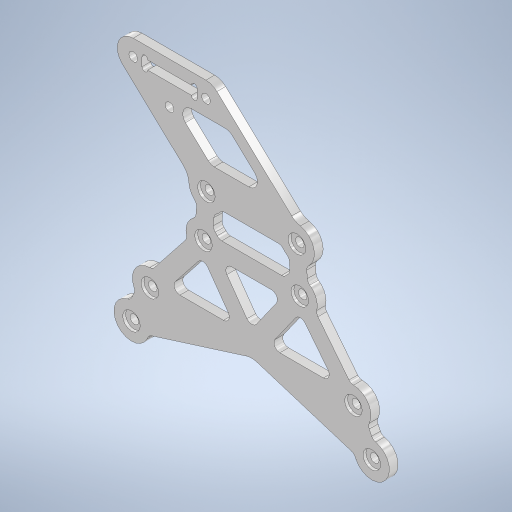
# Autodesk Inventor part: 中間ユニット外(shin)
Saved by Autodesk Inventor 2023 (Build 270158030, 158C)
## iProperties
Created: 2022-05-12
Part Number: 中間ユニット外(shin)
Material: アルミニウム 2014-T6
Document SubType Name: Modeling
Designer: muzho
Density: 2.78927 g/cm^3
Appearance: サテン
Author: muzho
Autodesk Inventor part; units mm, degrees
ref_plane "YZ Plane" through (0, 0, 0) normal (1, 0, 0) x (0, 1, 0)
ref_plane "XZ Plane" through (0, 0, 0) normal (0, 1, 0) x (-1, 0, 0)
ref_plane "XY Plane" through (0, 0, 0) normal (0, 0, 1) x (1, 0, 0)
sketch "スケッチ1" plane through (0, 0, 0) normal (0, 0, 1) x (1, 0, 0)
  circle A0 centre (-15.5646, 38.363) radius 1.5
  circle A1 centre (-15.5646, 38.363) radius 3.025
  circle A2 centre (-16.5506, 23.3453) radius 1.5
  circle A3 centre (-16.5506, 23.3453) radius 3.025
  circle A4 centre (-35, 0) radius 1.5
  circle A5 centre (-35, 0) radius 3.025
  circle A6 centre (-41.3199, -13) radius 1.5
  circle A7 centre (-41.3199, -13) radius 3.025
  circle A8 centre (41.3199, -13) radius 1.5
  circle A9 centre (41.3199, -13) radius 3.025
  circle A10 centre (35, 0) radius 3.025
  circle A11 centre (35, 0) radius 1.5
  circle A12 centre (16.5506, 23.3453) radius 3.025
  circle A13 centre (16.5506, 23.3453) radius 1.5
  circle A14 centre (15.5646, 38.363) radius 3.025
  circle A15 centre (15.5646, 38.363) radius 1.5
  circle A16 centre (-15.5646, 38.363) radius 6.025
  circle A17 centre (-16.5506, 23.3453) radius 6.025
  circle A18 centre (-35, 0) radius 6.025
  circle A19 centre (-41.3199, -13) radius 6.025
  circle A20 centre (15.5646, 38.363) radius 6.025
  circle A21 centre (16.5506, 23.3453) radius 6.025
  circle A22 centre (35, 0) radius 6.025
  circle A23 centre (41.3199, -13) radius 6.025
  line L0 (15.5646, 38.363) -> (16.5506, 23.3453) construction
  line L1 (16.5506, 23.3453) -> (35, 0) construction
  line L2 (35, 0) -> (41.3199, -13) construction
  line L3 (12.9134, 32.9527) -> (13.2147, 28.3626)
  line L4 (18.9005, 33.3458) -> (19.2019, 28.7557)
  line L5 (17.4366, 17.3858) -> (28.8054, 3)
  line L6 (22.144, 21.106) -> (34.114, 5.9595)
  line L7 (39.9825, -3.3875) -> (41.7335, -6.9892)
  line L8 (15.5646, 38.363) -> (0, 38.363) construction
  line L9 (16.5506, 23.3453) -> (0, 23.3453) construction
  line L10 (16.5506, 23.3453) -> (0, 0) construction
  line L11 (0, 0) -> (35, 0) construction
  line L12 (41.3199, -13) -> (0, 0) construction
  line L13 (10.3396, 41.363) -> (0, 41.363)
  line L14 (10.3396, 35.363) -> (0, 35.363)
  line L15 (11.3256, 26.3453) -> (0, 26.3453)
  line L16 (10.7463, 20.3453) -> (0, 20.3453)
  line L17 (10.7463, 20.3453) -> (-0.0011, 5.1857)
  line L18 (15.9761, 17.3478) -> (5.8043, 3)
  line L19 (5.8043, 3) -> (28.8054, 3)
  line L20 (28.8054, 3) -> (29.4066, 2.2393) construction
  line L21 (28.8054, 3) -> (29.775, 3) construction
  line L22 (29.5814, -2.6342) -> (35.9013, -15.6342)
  line L23 (29.7592, -3) -> (19.5315, -3)
  line L24 (19.5315, -3) -> (31.606, -6.7989)
  line L25 (1.8007, -3.7115) -> (35.216, -14.2246)
  line L26 (0, 0) -> (0, 9.2146) construction
  line L27 (-10.3396, 41.363) -> (0, 41.363)
  line L28 (-10.3396, 35.363) -> (0, 35.363)
  line L29 (-11.3256, 26.3453) -> (0, 26.3453)
  line L30 (-10.7463, 20.3453) -> (0, 20.3453)
  line L31 (-12.9134, 32.9527) -> (-13.2147, 28.3626)
  line L32 (-18.9005, 33.3458) -> (-19.2019, 28.7557)
  line L33 (-10.7463, 20.3453) -> (0.0011, 5.1857)
  line L34 (-15.9761, 17.3478) -> (-5.8043, 3)
  line L35 (-17.4366, 17.3858) -> (-28.8054, 3)
  line L36 (-22.144, 21.106) -> (-34.114, 5.9595)
  line L37 (-5.8043, 3) -> (-28.8054, 3)
  line L38 (-29.7592, -3) -> (-19.5315, -3)
  line L39 (-19.5315, -3) -> (-31.606, -6.7989)
  line L40 (-29.5814, -2.6342) -> (-35.9013, -15.6342)
  line L41 (-39.9825, -3.3875) -> (-41.7335, -6.9892)
  line L42 (-1.8007, -3.7115) -> (-35.216, -14.2246)
  arc A24 (1.8007, -3.7115) -> (-1.8007, -3.7115) centre (0, -9.4349) ccw
  point P0 (0, 5.1872)
  point P1 (-35.9013, -15.6342)
  point P2 (0, -3.145)
  dimension "d0" = 3
  dimension "d1" = 3
  dimension "d2" = 3
  dimension "d3" = 3
  dimension "d4" = 3
  dimension "d5" = 3
  dimension "d6" = 3
  dimension "d7" = 3
  dimension "d8" = 6
  dimension "d9" = 3
  dimension "d10" = 6
  dimension "d11" = 3
  dimension "d12" = 6
  dimension "d13" = 3
  dimension "d14" = 6
  dimension "d15" = 3
  dimension "d16" = 6
  dimension "d17" = 3
  dimension "d18" = 3
  dimension "d19" = 3
  dimension "d20" = 6
  dimension "d21" = 3
  dimension "d22" = 3
  dimension "d57" = 6
  constraints: 88 end point, 25 centre point, 24 symmetric about line, 19 point on circle, 10 horizontal, 10 parallel, 6 point on line, 3 tangent, 1 vertical, 25 other
  measures "d0" radial gap between concentric circles of A1 A16
  measures "d1" radial gap between concentric circles of A3 A17
  measures "d2" radial gap between concentric circles of A5 A18
  measures "d3" radial gap between concentric circles of A7 A19
  measures "d4" radial gap between concentric circles of A14 A20
  measures "d5" radial gap between concentric circles of A12 A21
  measures "d6" radial gap between concentric circles of A10 A22
  measures "d7" radial gap between concentric circles of A9 A23
  measures "d8" distance between parallel lines of L3 L4
  measures "d9" distance between parallel lines of L3 L0
  measures "d10" distance between parallel lines of L5 L6
  measures "d11" distance between parallel lines of L5 L1
  measures "d12" distance between parallel lines of L14 L13
  measures "d13" distance between parallel lines of L14 L8
  measures "d14" distance between parallel lines of L16 L15
  measures "d15" distance between parallel lines of L16 L9
  measures "d16" distance between parallel lines of L18 L17
  measures "d17" distance between parallel lines of L17 L10
  measures "d18" distance between parallel lines of L11 L19
  measures "d19" distance between parallel lines of L2 L7
  measures "d20" distance between parallel lines of L19 L23
  measures "d21" distance between parallel lines of L12 L24
  measures "d22" distance between parallel lines of L25 L12
  measures "d57" radius of A24
extrude "押し出し1" add sketch "スケッチ1" along normal blind 3 contours A16 | A16 L27 L13 A20 L14 L28 | A16 L31 A17 L32 | A17 | A20 | A17 L35 L37 L34 L29 L15 A21 L18 L19 L5 L6 A22 L22 L23 L24 L25 A24 L42 L40 L39 L38 A18 L36 | A20 L4 A21 L3 | A18 | A21 | A18 L40 A19 L41 | A19 | L38 L39 L40 | A22 | A22 L7 A23 L22 | L22 L24 L23 | A23
extrude "押し出し2" add sketch "スケッチ1" along normal blind 2 contours A1 | A3 | A5 | A7 | A9 | A10 | A12 | A14
fillet "フィレット1" radius 2 35 edges at (-13.2147, 28.3626, 1.5) (-11.3256, 26.3453, 1.5) (-12.9134, 32.9527, 1.5) (-10.3396, 35.363, 1.5) (13.2147, 28.3626, 1.5) (12.9134, 32.9527, 1.5) (11.3256, 26.3453, 1.5) (10.3396, 35.363, 1.5) (-10.3396, 41.363, 1.5) (10.3396, 41.363, 1.5) (18.9005, 33.3458, 1.5) (19.2019, 28.7557, 1.5) (22.144, 21.106, 1.5) (39.9825, -3.3875, 1.5) (34.114, 5.9595, 1.5) (35.216, -14.2246, 1.5) (-35.216, -14.2246, 1.5) (-39.9825, -3.3875, 1.5) (-41.7335, -6.9892, 1.5) (-34.114, 5.9595, 1.5) (-22.144, 21.106, 1.5) (-19.2019, 28.7557, 1.5) (-18.9005, 33.3458, 1.5) (-5.8043, 3, 1.5) (0, 5.1872, 1.5) (5.8043, 3, 1.5) (-28.8054, 3, 1.5) (28.8054, 3, 1.5) (10.7463, 20.3453, 1.5) (-10.7463, 20.3453, 1.5) (-17.4366, 17.3858, 1.5) (-15.9761, 17.3478, 1.5) (15.9761, 17.3478, 1.5) (17.4366, 17.3858, 1.5) (41.7335, -6.9892, 1.5)
sketch "スケッチ2" plane through (0, 0, 0) normal (0, 0, -1) x (-1, 0, 0)
  arc A0 (-10.852, 42.1169) -> (-19.6192, 33.9064) centre (-15.5646, 38.363) ccw projected
  arc A1 (-16.7318, 44.2739) -> (-13.7829, 45.7901) centre (-17.8942, 50.1602) ccw
  line L0 (-13.7829, 45.7901) -> (11.9431, 69.9924)
  line L1 (19.7118, 81.8816) -> (-21.6862, 42.9356) construction
  arc A2 (-10.852, 42.1169) -> (-19.6192, 33.9064) centre (-15.5646, 38.363) ccw projected
  line L2 (15.7118, 71.4865) -> (40.7118, 71.4865)
  line L3 (44.4804, 61.9806) -> (23.4671, 42.2119)
  arc A3 (23.4671, 42.2119) -> (21.584, 38.1019) centre (27.5783, 37.8418) ccw
  arc A4 (19.6192, 33.9064) -> (10.852, 42.1169) centre (15.5646, 38.363) ccw projected
  arc A5 (15.7118, 71.4865) -> (11.9431, 69.9924) centre (15.7118, 65.9865) ccw
  arc A6 (44.4804, 61.9806) -> (40.7118, 71.4865) centre (40.7118, 65.9865) ccw
  arc A7 (-10.852, 42.1169) -> (-9.2876, 41.363) centre (-9.2876, 43.363) ccw projected
  line L4 (-9.2876, 41.363) -> (9.2876, 41.363) projected
  arc A8 (9.2876, 41.363) -> (10.852, 42.1169) centre (9.2876, 43.363) ccw projected
  line L5 (6.8101, 59.6715) -> (-1.0679, 52.2601)
  arc A9 (8.8657, 60.4865) -> (6.8101, 59.6715) centre (8.8657, 57.4865) ccw
  line L6 (8.8657, 60.4865) -> (20.7172, 60.4865)
  arc A10 (22.7728, 55.3014) -> (20.7172, 60.4865) centre (20.7172, 57.4865) ccw
  line L7 (22.7728, 55.3014) -> (14.8948, 47.89)
  arc A11 (-1.0679, 52.2601) -> (0.9877, 47.0751) centre (0.9877, 50.0751) ccw
  line L8 (0.9877, 47.0751) -> (12.8392, 47.0751)
  arc A12 (12.8392, 47.0751) -> (14.8948, 47.89) centre (12.8392, 50.0751) ccw
  line L9 (18.8039, 63.4865) -> (21.0041, 63.4865)
  arc A13 (24.3649, 52.7226) -> (24.8918, 61.796) centre (20.7172, 57.4865) ccw
  arc A14 (9.3776, 45.1743) -> (15.0189, 44.485) centre (12.8392, 50.0751) ccw construction
  circle A15 centre (40.7118, 65.9865) radius 1.5 projected
  circle A16 centre (15.7118, 65.9865) radius 1.5 projected
  circle A17 centre (15.7118, 65.9865) radius 1.5 projected
  circle A18 centre (28.2118, 57.2015) radius 1.5 projected
  line L10 (30.7118, 64.4865) -> (25.7118, 64.4865) projected
  line L11 (28.2118, 65.7583) -> (28.2118, 63.0037)
  line L12 (25.7118, 64.4865) -> (20.7118, 64.4865)
  line L13 (30.7118, 64.4865) -> (35.7118, 64.4865)
  arc A19 (35.7118, 64.4865) -> (37.7118, 64.4865) centre (36.7118, 64.4865) ccw
  line L14 (37.7118, 64.4865) -> (37.7118, 67.4865)
  arc A20 (37.7118, 67.4865) -> (35.7118, 67.4865) centre (36.7118, 67.4865) ccw
  line L15 (35.7118, 67.4865) -> (20.7118, 67.4865)
  arc A21 (18.7118, 64.4865) -> (20.7118, 64.4865) centre (19.7118, 64.4865) ccw
  line L16 (18.7118, 64.4865) -> (18.7118, 67.4865)
  arc A22 (20.7118, 67.4865) -> (18.7118, 67.4865) centre (19.7118, 67.4865) ccw
  line L17 (0, 41.363) -> (0, 67.4865) construction
  arc A23 (13.7829, 45.7901) -> (16.7318, 44.2739) centre (17.8942, 50.1602) ccw construction
  line L18 (13.7829, 45.7901) -> (-11.9431, 69.9924) construction
  line L19 (-15.7118, 71.4865) -> (-40.7118, 71.4865) construction
  line L20 (-44.4804, 61.9806) -> (-23.4671, 42.2119) construction
  arc A24 (-21.584, 38.1019) -> (-23.4671, 42.2119) centre (-27.5783, 37.8418) ccw construction
  arc A25 (-11.9431, 69.9924) -> (-15.7118, 71.4865) centre (-15.7118, 65.9865) ccw construction
  arc A26 (-40.7118, 71.4865) -> (-44.4804, 61.9806) centre (-40.7118, 65.9865) ccw construction
  line L21 (-6.8101, 59.6715) -> (1.0679, 52.2601) construction
  arc A27 (-6.8101, 59.6715) -> (-8.8657, 60.4865) centre (-8.8657, 57.4865) ccw construction
  line L22 (-8.8657, 60.4865) -> (-20.7172, 60.4865) construction
  arc A28 (-20.7172, 60.4865) -> (-22.7728, 55.3014) centre (-20.7172, 57.4865) ccw construction
  line L23 (-22.7728, 55.3014) -> (-14.8948, 47.89) construction
  arc A29 (-0.9877, 47.0751) -> (1.0679, 52.2601) centre (-0.9877, 50.0751) ccw construction
  line L24 (-0.9877, 47.0751) -> (-12.8392, 47.0751) construction
  arc A30 (-14.8948, 47.89) -> (-12.8392, 47.0751) centre (-12.8392, 50.0751) ccw construction
  line L25 (-18.8039, 63.4865) -> (-21.0041, 63.4865) construction
  circle A31 centre (-40.7118, 65.9865) radius 1.5 construction
  circle A32 centre (-15.7118, 65.9865) radius 1.5 construction
  circle A33 centre (-15.7118, 65.9865) radius 1.5 construction
  circle A34 centre (-28.2118, 57.2015) radius 1.5 construction
  line L26 (-30.7118, 64.4865) -> (-25.7118, 64.4865) construction
  line L27 (-28.2118, 65.7583) -> (-28.2118, 63.0037) construction
  line L28 (-25.7118, 64.4865) -> (-20.7118, 64.4865) construction
  line L29 (-30.7118, 64.4865) -> (-35.7118, 64.4865) construction
  arc A35 (-37.7118, 64.4865) -> (-35.7118, 64.4865) centre (-36.7118, 64.4865) ccw construction
  line L30 (-37.7118, 64.4865) -> (-37.7118, 67.4865) construction
  arc A36 (-35.7118, 67.4865) -> (-37.7118, 67.4865) centre (-36.7118, 67.4865) ccw construction
  line L31 (-35.7118, 67.4865) -> (-20.7118, 67.4865) construction
  arc A37 (-18.7118, 67.4865) -> (-20.7118, 67.4865) centre (-19.7118, 67.4865) ccw construction
  arc A38 (-20.7118, 64.4865) -> (-18.7118, 64.4865) centre (-19.7118, 64.4865) ccw construction
  line L32 (-18.7118, 64.4865) -> (-18.7118, 67.4865) construction
  point P0 (0, 0)
  point P1 (28.2118, 64.4865)
  point P2 (-28.2118, 64.4865)
  point P3 (16.7318, 44.2739)
  dimension "d28" = 6
  dimension "d33" = 6
  dimension "d37" = 3
  dimension "d38" = 3
  dimension "d39" = 3
  dimension "d40" = 3
  dimension "d42" = 3
  dimension "d43" = 3
  dimension "d44" = 4
  dimension "d45" = 4
  dimension "d47" = 1
  dimension "d48" = 3
  dimension "d49" = 1
  dimension "d50" = 19
  dimension "d51" = 3
  dimension "d52" = 3
  constraints: 60 end point, 56 point on circle, 54 symmetric about line, 30 centre point, 20 tangent, 6 horizontal, 4 parallel, 4 point on line, 3 concentric, 3 vertical, 2 coincident, 2 line through centre, 2 midpoint, 18 other
  measures "d28" radius of A1
  measures "d33" radius of A3
  measures "d37" radius of A9
  measures "d38" radius of A10
  measures "d39" radius of A11
  measures "d40" radius of A12
  measures "d42" radial gap between concentric circles of A10 A13
  measures "d43" radial gap between concentric circles of A14 A12
  measures "d44" distance between parallel lines of L0 L5
  measures "d45" radial gap between concentric circles of A16 A5
  measures "d47" radius of A19
  measures "d48" distance of L14.start L14.end
  measures "d49" radius of A20
  measures "d50" distance between parallel lines of L14 L16
  measures "d51" distance between parallel lines of L12 L15
  measures "d52" distance between parallel lines of L6 L9
extrude "押し出し5" add sketch "スケッチ2" against normal blind 3
equation "\"d9\" = 0.5 * d8"
equation "\"d11\" = 0.5 * d10"
equation "\"d13\" = 0.5 * d12"
equation "\"d15\" = 0.5 * d14"
equation "\"d17\" = 0.5 * d16"
equation "\"d18\" = 0.5 * d20"
